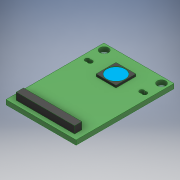
# Autodesk Inventor part: Module_ArducamMini-Rev
Saved by Autodesk Inventor 2017 (Build 210142000, 142)
## iProperties
Created: 2018-01-06
Part Number: Module_ArducamMini-Rev
Material: Epoxy Resin
Document SubType Name: Modeling
Designer: Bradley
Density: 1.14 g/cm^3
Appearance: Smooth - Dark Forest Green
Mass: 1.66546 g
Surface Area: 20.0013 cm^2
Volume: 1.46093 cm^3
Author: Bradley
Autodesk Inventor part; units mm, degrees
ref_plane "YZ Plane" through (0, 0, 0) normal (1, 0, 0) x (0, 1, 0)
ref_plane "XZ Plane" through (0, 0, 0) normal (0, 1, 0) x (-1, 0, 0)
ref_plane "XY Plane" through (0, 0, 0) normal (0, 0, 1) x (1, 0, 0)
sketch "Sketch1" plane through (0, 0, 0) normal (0, 0, 1) x (1, 0, 0)
  line L0 (-12.2, -17.05) -> (12.2, -17.05)
  line L1 (12.2, -17.05) -> (12.2, 17.05)
  line L2 (12.2, 17.05) -> (-12.2, 17.05)
  line L3 (-12.2, 17.05) -> (-12.2, -17.05)
  line L4 (-12.2, -17.05) -> (12.2, 17.05) construction
  line L5 (12.2, -17.05) -> (-12.2, 17.05) construction
  circle A0 centre (-10, 14.92) radius 1.5
  circle A1 centre (10, 14.92) radius 1.5
  line L6 (-10, 14.92) -> (10, 14.92) construction
  circle A2 centre (-9, 9.05) radius 0.8
  circle A3 centre (-10, 9.05) radius 0.8
  circle A4 centre (9, 9.05) radius 0.8
  circle A5 centre (10, 9.05) radius 0.8
  line L7 (-9, 9.05) -> (9, 9.05) construction
  line L8 (-10, 9.05) -> (10, 9.05) construction
  point P0 (0, 0)
  point P1 (0, 9.05)
  point P2 (0, 14.92)
  point P3 (0, 0)
  point P4 (0, 0)
  dimension "d0" = 24.4
  dimension "d1" = 34.1
  dimension "d2" = 2.13
  dimension "d3" = 3
  dimension "d4" = 10
  dimension "d13" = 20
  dimension "d14" = 18
  dimension "d15" = 1.6
  dimension "d16" = 8
  constraints: 18 end point, 7 midpoint, 6 centre point, 4 equal radius, 4 horizontal, 2 parallel, 2 vertical alignment, 1 horizontal alignment, 1 perpendicular
  measures "d0" distance of L2.end L1.end
  measures "d1" distance of L1.end L0.end
  measures "d2" distance from line of L2 L6.start
  measures "d3" diameter of A0
  measures "d4" horizontal distance of point (0, 0) L6.start
  measures "d13" distance of L8.start L8.end
  measures "d14" distance of L7.start L7.end
  measures "d15" diameter of A3
  measures "d16" distance between parallel lines of L2 L7
extrude "Extrusion1" add sketch "Sketch1" along normal mid plane 1.6
sketch "Sketch2" plane through (0, 0, -0.8) normal (0, 0, -1) x (-1, 0, 0)
  circle A0 centre (-10, 14.92) radius 1.5 projected
  circle A1 centre (10, 14.92) radius 1.5 projected
  line L0 (-12.2, -17.05) -> (12.2, -17.05) projected
  line L1 (12.2, -17.05) -> (12.2, 17.05) projected
  line L2 (12.2, 17.05) -> (-12.2, 17.05) projected
  line L3 (-12.2, 17.05) -> (-12.2, -17.05) projected
  line L4 (-10.16, -12.99) -> (10.16, -12.99)
  line L5 (10.16, -12.99) -> (10.16, -15.53)
  line L6 (10.16, -15.53) -> (-10.16, -15.53)
  line L7 (-10.16, -15.53) -> (-10.16, -12.99)
  point P0 (0, 0)
  point P1 (0, -12.99)
  point P2 (-10.16, -14.26)
  dimension "d8" = 2.54
  dimension "d9" = 20.32
  dimension "d10" = 2.79
  constraints: 8 end point, 2 midpoint, 2 parallel, 1 horizontal, 1 perpendicular, 1 vertical alignment
  measures "d8" distance of L4.end L5.end
  measures "d9" distance of L4.start L4.end
  measures "d10" distance from line of L0 point (-10.16, -14.26)
extrude "Extrusion2" add sketch "Sketch2" against normal blind 4.1 contours L4 L5 L6 L7
sketch "Sketch3" plane through (0, 0, 0.8) normal (0, 0, 1) x (1, 0, 0)
  circle A0 centre (10, 14.92) radius 1.5 projected
  circle A1 centre (-10, 14.92) radius 1.5 projected
  arc A2 (-9.5, 8.4255) -> (-9.5, 9.6745) centre (-9, 9.05) ccw projected
  arc A3 (-9.5, 9.6745) -> (-9.5, 8.4255) centre (-10, 9.05) ccw projected
  line L0 (-12.2, -17.05) -> (12.2, -17.05) projected
  line L1 (12.2, -17.05) -> (12.2, 17.05) projected
  line L2 (12.2, 17.05) -> (-12.2, 17.05) projected
  line L3 (-12.2, 17.05) -> (-12.2, -17.05) projected
  arc A4 (9.5, 9.6745) -> (9.5, 8.4255) centre (9, 9.05) ccw projected
  arc A5 (9.5, 8.4255) -> (9.5, 9.6745) centre (10, 9.05) ccw projected
  line L4 (-3.4725, 12.5225) -> (3.4725, 12.5225)
  line L5 (3.4725, 12.5225) -> (3.4725, 5.5775)
  line L6 (3.4725, 5.5775) -> (-3.4725, 5.5775)
  line L7 (-3.4725, 5.5775) -> (-3.4725, 12.5225)
  point P0 (0, 0)
  point P1 (3.4725, 9.05)
  point P2 (0, 12.5225)
  dimension "d17" = 6.945
  constraints: 8 end point, 2 midpoint, 2 parallel, 2 perpendicular, 1 horizontal, 1 horizontal alignment, 1 vertical alignment
  measures "d17" distance of L4.start L4.end
extrude "Extrusion3" add sketch "Sketch3" along normal blind 0.78 contours L4 L5 L6 L7
sketch "Sketch4" plane through (0, 0, 1.58) normal (0, 0, 1) x (1, 0, 0)
  line L0 (3.4725, 12.5225) -> (-3.4725, 12.5225) projected
  line L1 (-3.4725, 12.5225) -> (-3.4725, 5.5775) projected
  line L2 (-3.4725, 5.5775) -> (3.4725, 5.5775) projected
  line L3 (3.4725, 5.5775) -> (3.4725, 12.5225) projected
  circle A0 centre (0, 9.05) radius 3.175
  point P0 (0, 0)
  point P1 (0, 12.5225)
  point P2 (-3.4725, 9.05)
  dimension "d20" = 6.35
  constraints: 2 midpoint, 1 centre point, 1 horizontal alignment, 1 vertical alignment
  measures "d20" diameter of A0
extrude "Extrusion4" cut sketch "Sketch4" against normal blind 0.1 contours A0
equation "\"d9\" = 8 * d8"
body "Solid1"
